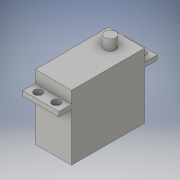
# Autodesk Inventor part: RTS Motor
Saved by Autodesk Inventor 2016 (Build 200138000, 138)
## iProperties
Created: 2016-10-05
Part Number: RTS Motor
Material: Generic
Document SubType Name: Modeling
Designer: MHSLibrary
Density: 1 g/cm^3
Appearance: Default
Author: MHSLibrary
Autodesk Inventor part; units mm, degrees
ref_plane "YZ Plane" through (0, 0, 0) normal (1, 0, 0) x (0, 1, 0)
ref_plane "XZ Plane" through (0, 0, 0) normal (0, 1, 0) x (-1, 0, 0)
ref_plane "XY Plane" through (0, 0, 0) normal (0, 0, 1) x (1, 0, 0)
sketch "Sketch1" plane through (0, 0, 0) normal (0, 0, 1) x (1, 0, 0)
  line L0 (-7.4537, 7.1113) -> (12.5361, 7.1113)
  line L1 (12.5361, 7.1113) -> (12.5361, -28.8297)
  line L2 (12.5361, -28.8297) -> (-7.4537, -28.8297)
  line L3 (-7.4537, -28.8297) -> (-7.4537, 7.1113)
  point P0 (0, 0)
  dimension "d0" = 19.9898
  dimension "d1" = 35.941
  constraints: 8 end point, 2 parallel, 1 horizontal, 1 perpendicular
  measures "d0" distance of L0.start L0.end
  measures "d1" distance of L0.end L1.end
extrude "Extrusion1" add sketch "Sketch1" along normal blind 40.386
sketch "Sketch2" plane through (0, 0, 0) normal (0, 0, -1) x (-1, 0, 0)
  line L0 (-12.5361, -28.8297) -> (-12.5361, 7.1113) projected
  line L1 (7.4537, -28.8297) -> (7.4537, 7.1113) projected
  line L2 (-12.5361, 0.4311) -> (7.4537, 0.4311)
  line L3 (7.4537, 0.4311) -> (7.4537, -2.1597)
  line L4 (7.4537, -2.1597) -> (-12.5361, -2.1597)
  line L5 (-12.5361, -2.1597) -> (-12.5361, 0.4311)
  line L6 (7.4537, 7.1113) -> (-12.5361, 7.1113) projected
  line L7 (-12.5361, -28.8297) -> (7.4537, -28.8297) projected
  line L8 (7.4537, 7.1113) -> (7.4537, -28.8297) projected
  line L9 (7.4537, 0.4311) -> (-12.5361, 0.4311)
  line L10 (-12.5361, 0.4311) -> (-12.5361, -2.1597)
  line L11 (-12.5361, -2.1597) -> (7.4537, -2.1597)
  line L12 (7.4537, -2.1597) -> (7.4537, 0.4311)
  point P0 (0, 0)
  dimension "d4" = 6.6802
  dimension "d5" = 2.5908
  dimension "d6" = 26.67
  dimension "d7" = 19.9898
  dimension "d8" = 2.5908
  constraints: 16 end point, 4 parallel, 3 point on line, 2 horizontal, 2 perpendicular
  measures "d4" distance between parallel lines of L2 L6
  measures "d5" distance between parallel lines of L4 L2
  measures "d6" distance between parallel lines of L7 L4
  measures "d7" distance between parallel lines of L3 L5
  measures "d8" distance between parallel lines of L4 L9
extrude "Extrusion2" add sketch "Sketch2" along normal blind 7.0104 contours L0 L2 L1 L4
sketch "Sketch3" plane through (0, 0, 40.386) normal (0, 0, 1) x (1, 0, 0)
  point P0 (0, 0)
sketch "Sketch4" plane through (0, 0, 40.386) normal (0, 0, 1) x (1, 0, 0)
  line L0 (-7.4537, -2.1597) -> (-7.4537, 0.4311) projected
  line L1 (12.5361, -2.1597) -> (-7.4537, -2.1597) projected
  line L2 (-7.4537, 0.4311) -> (12.5361, 0.4311)
  line L3 (12.5361, 0.4311) -> (12.5361, -2.1597)
  line L4 (12.5361, -2.1597) -> (-7.4537, -2.1597)
  line L5 (-7.4537, -2.1597) -> (-7.4537, 0.4311)
  point P0 (0, 0)
  constraints: 8 end point, 2 parallel, 1 horizontal, 1 perpendicular
extrude "Extrusion3" add sketch "Sketch4" along normal blind 7.0104
sketch "Sketch5" plane through (-7.4537, 0.4311, 40.386) normal (0, 1, 0) x (1, 0, 0)
  circle A0 centre (14.9098, -3.3973) radius 2.2479
  line L0 (19.9898, 0) -> (19.9898, -7.0104) projected
  circle A1 centre (5.08, -3.5052) radius 2.2479
  line L1 (0, 0) -> (0, -7.0104) projected
  point P0 (7.4537, 40.386)
  dimension "d13" = 5.08
  dimension "d14" = 5.08
  dimension "d15" = 4.4958
  dimension "d16" = 4.4958
  dimension "d17" = 5.3346
  constraints: 2 centre point
  measures "d13" distance from line of L0 A0.centre
  measures "d14" distance from line of L1 A1.centre
  measures "d15" diameter of A1
  measures "d16" diameter of A0
sketch "Sketch6" plane through (-7.4537, 7.1113, 0) normal (0, 1, 0) x (1, 0, 0)
  point P0 (7.4537, 0)
sketch "Sketch7" plane through (-7.4537, 0.4311, 0) normal (0, 1, 0) x (1, 0, 0)
  circle A0 centre (14.9098, 3.6831) radius 2.2479
  circle A1 centre (5.08, 3.6831) radius 2.2479
  line L0 (19.9898, 0) -> (19.9898, 7.0104) projected
  line L1 (0, 0) -> (0, 7.0104) projected
  point P0 (7.4537, 0)
  dimension "d18" = 5.08
  dimension "d19" = 5.08
  dimension "d20" = 4.4958
  dimension "d21" = 4.4958
  dimension "d22" = 5.334
  constraints: 2 centre point
  measures "d18" distance from line of L0 A0.centre
  measures "d19" distance from line of L1 A1.centre
  measures "d20" diameter of A0
  measures "d21" diameter of A1
hole "Hole1" at (7.4561, 0.4311, 43.7833) at (-2.3737, 0.4311, 43.8912) direction (0, -1, 0) diameter 4.4958 end through all
hole "Hole2" at (7.4561, 0.4311, -3.6831) at (-2.3737, 0.4311, -3.6831) direction (0, -1, 0) diameter 4.4958 end through all
sketch "Sketch8" plane through (-7.4537, 7.1113, 0) normal (0, 1, 0) x (1, 0, 0)
  circle A0 centre (9.9711, -8.9281) radius 2.9845
  line L0 (0, 0) -> (19.9898, 0) projected
  point P0 (7.4537, 0)
  dimension "d37" = 5.9436
  dimension "d38" = 5.969
  constraints: 1 centre point
  measures "d37" distance edge to line of A0 L0
  measures "d38" diameter of A0
extrude "Extrusion4" add sketch "Sketch8" along normal blind 5.9944
sketch "Sketch9" plane through (0, 0, 0) normal (0, 0, -1) x (-1, 0, 0)
  point P0 (0, 0)
sketch "Sketch10" plane through (-7.4537, 7.1113, 0) normal (0, 1, 0) x (1, 0, 0)
  line L0 (0, 0) -> (19.9898, 0) projected
  line L1 (19.9898, 0) -> (19.9898, -40.386) projected
  line L2 (0, 0) -> (0, -40.386) projected
  line L3 (19.9898, -40.386) -> (0, -40.386) projected
  circle A0 centre (14.9098, -43.7833) radius 2.2479 projected
  circle A1 centre (5.08, -43.8912) radius 2.2479 projected
  circle A2 centre (14.9098, 3.6831) radius 2.2479 projected
  circle A3 centre (5.08, 3.6831) radius 2.2479 projected
  point P0 (7.4537, 0)
body "Solid1"
